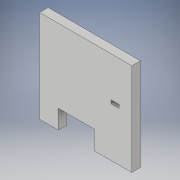
# Autodesk Inventor part: front
Saved by Autodesk Inventor 2019 (Build 230136000, 136)
## iProperties
Created: 2019-12-08
Part Number: front
Material: Generic
Document SubType Name: Modeling
Designer: HP
Density: 1 g/cm^3
Appearance: Default
Author: HP
Autodesk Inventor part; units mm, degrees
ref_plane "YZ Plane" through (0, 0, 0) normal (1, 0, 0) x (0, 1, 0)
ref_plane "XZ Plane" through (0, 0, 0) normal (0, 1, 0) x (-1, 0, 0)
ref_plane "XY Plane" through (0, 0, 0) normal (0, 0, 1) x (1, 0, 0)
sketch "Sketch1" plane through (0, 0, 0) normal (0, 0, 1) x (1, 0, 0)
  point P0 (0, 0)
sketch "Sketch2" plane through (0, 0, 0) normal (0, 0, 1) x (1, 0, 0)
  line L0 (0, 0) -> (10.9474, 0)
  line L1 (10.9474, 0) -> (10.9474, 10.9728)
  line L2 (10.9474, 10.9728) -> (0, 10.9728)
  line L3 (0, 10.9728) -> (0, 0)
  dimension "d0" = 10.9474
  dimension "d1" = 10.9728
  constraints: 8 end point, 2 parallel, 1 horizontal, 1 perpendicular
  measures "d0" distance of L2.end L1.end
  measures "d1" distance of L1.end L0.end
extrude "Extrusion1" add sketch "Sketch2" along normal blind 1.016
sketch "Sketch3" plane through (0, 0, 1.016) normal (0, 0, 1) x (1, 0, 0)
  line L0 (0, 0) -> (10.9474, 0) projected
  line L1 (2.2167, 0) -> (6.4763, 0)
  line L2 (6.4763, 0) -> (6.4763, 2.2384)
  line L3 (6.4763, 2.2384) -> (2.2167, 2.2384)
  line L4 (2.2167, 2.2384) -> (2.2167, 0)
  line L5 (8.5191, 6.2372) -> (9.3015, 6.2372)
  line L6 (9.3015, 6.2372) -> (9.3015, 5.7591)
  line L7 (9.3015, 5.7591) -> (8.5191, 5.7591)
  line L8 (8.5191, 5.7591) -> (8.5191, 6.2372)
  constraints: 16 end point, 4 parallel, 2 horizontal, 2 perpendicular, 1 point on line
extrude "Extrusion2" cut sketch "Sketch3" against normal blind 1.016 contours L4 L3 L2 L0
sketch "Sketch4" plane through (0, 0, 1.016) normal (0, 0, 1) x (1, 0, 0)
  line L0 (8.4757, 6.2372) -> (9.4319, 6.2372)
  line L1 (9.4319, 6.2372) -> (9.4319, 5.846)
  line L2 (9.4319, 5.846) -> (8.4757, 5.846)
  line L3 (8.4757, 5.846) -> (8.4757, 6.2372)
  point P0 (0, 0)
  constraints: 8 end point, 2 parallel, 1 horizontal, 1 perpendicular
extrude "Extrusion3" cut sketch "Sketch4" against normal blind 1.016
body "Solid1"
